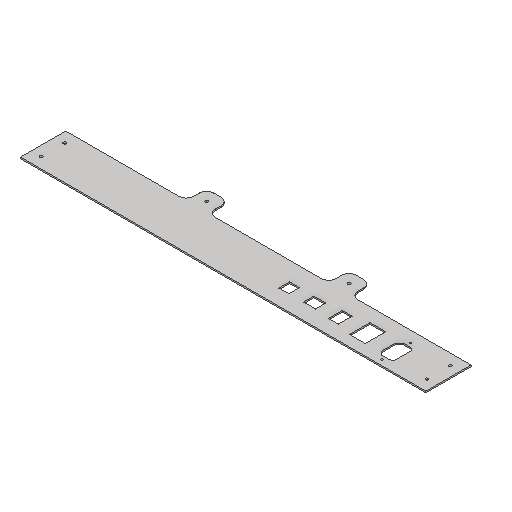
# Autodesk Inventor part: LC_ALU_2mm_Back_Plate
Saved by Autodesk Inventor 2026.1 (Build 301233000, 233)
## iProperties
Created: 2016-06-26
Part Number: LC_ALU_2mm_Back_Plate
Material: Ogólny
Document SubType Name: Modeling
Designer: Andrzej
Density: 1 g/cm^3
Appearance: Obrobione — aluminium
Mass: 72.1532 g
Surface Area: 749.313 cm^2
Volume: 72.1532 cm^3
Author: Andrzej
Autodesk Inventor part; units mm, degrees
ref_plane "YZ Plane" through (0, 0, 0) normal (1, 0, 0) x (0, 1, 0)
ref_plane "XZ Plane" through (0, 0, 0) normal (0, 1, 0) x (-1, 0, 0)
ref_plane "XY Plane" through (0, 0, 0) normal (0, 0, 1) x (1, 0, 0)
sketch "Szkic1" plane through (0, 0, 0) normal (0, 0, 1) x (1, 0, 0)
  line L0 (-89.8533, 62.242) -> (466.1467, 62.242)
  line L1 (466.1467, 62.242) -> (466.1467, 0.242)
  line L2 (466.1467, 0.242) -> (-89.8533, 0.242)
  line L3 (-89.8533, 0.242) -> (-89.8533, 62.242)
  line L4 (75.48, 62.242) -> (105.48, 62.242)
  line L5 (105.48, 62.242) -> (105.48, 90.242)
  line L6 (105.48, 90.242) -> (75.48, 90.242)
  line L7 (75.48, 90.242) -> (75.48, 62.242)
  line L8 (270.8133, 62.242) -> (300.8133, 62.242)
  line L9 (300.8133, 62.242) -> (300.8133, 90.242)
  line L10 (300.8133, 90.242) -> (270.8133, 90.242)
  line L11 (270.8133, 90.242) -> (270.8133, 62.242)
  arc A0 (403.6467, 13.242) -> (407.6467, 17.242) centre (403.6467, 17.242) ccw
  line L12 (407.6467, 17.242) -> (407.6467, 37.242)
  arc A1 (407.6467, 37.242) -> (403.6467, 41.242) centre (403.6467, 37.242) ccw
  line L13 (388.647, 36.242) -> (393.647, 41.242)
  line L14 (388.647, 36.242) -> (388.647, 18.242)
  line L15 (393.647, 13.242) -> (388.647, 18.242)
  line L16 (393.647, 41.242) -> (403.6467, 41.242)
  line L17 (393.647, 13.242) -> (403.6467, 13.242)
  line L18 (393.4399, 41.742) -> (388.147, 36.4491)
  line L19 (388.147, 36.4491) -> (388.147, 18.0348)
  line L20 (388.147, 18.0348) -> (393.4399, 12.742)
  line L21 (393.4399, 12.742) -> (403.6467, 12.742)
  arc A2 (403.6467, 12.742) -> (408.1467, 17.242) centre (403.6467, 17.242) ccw
  line L22 (408.1467, 17.242) -> (408.1467, 37.242)
  arc A3 (408.1467, 37.242) -> (403.6467, 41.742) centre (403.6467, 37.242) ccw
  line L23 (403.6467, 41.742) -> (393.4399, 41.742)
  circle A4 centre (398.6468, 46.742) radius 1.5
  circle A5 centre (398.6467, 7.742) radius 1.5
  line L24 (346.447, 43.242) -> (368.147, 43.242)
  line L25 (368.147, 43.242) -> (368.147, 15.242)
  line L26 (368.147, 15.242) -> (346.447, 15.242)
  line L27 (346.447, 15.242) -> (346.447, 43.242)
  line L28 (276.447, 36.242) -> (292.947, 36.242)
  line L29 (292.947, 36.242) -> (292.947, 22.242)
  line L30 (292.947, 22.242) -> (276.447, 22.242)
  line L31 (276.447, 22.242) -> (276.447, 36.242)
  line L32 (242.947, 36.542) -> (256.447, 36.542)
  line L33 (256.447, 36.542) -> (256.447, 21.942)
  line L34 (256.447, 21.942) -> (242.947, 21.942)
  line L35 (242.947, 21.942) -> (242.947, 36.542)
  line L36 (312.947, 38.742) -> (326.447, 38.742)
  line L37 (326.447, 38.742) -> (326.447, 19.742)
  line L38 (326.447, 19.742) -> (312.947, 19.742)
  line L39 (312.947, 19.742) -> (312.947, 38.742)
  point P0 (90.48, 75.242)
  point P1 (285.8133, 75.242)
  point P2 (-76.3533, 47.242)
  point P3 (452.6467, 47.242)
  point P4 (-76.3533, 15.242)
  point P5 (452.6467, 15.242)
  dimension "d0" = 556
  dimension "d1" = 62
  dimension "d2" = 30
  dimension "d3" = 28
  dimension "d4" = 30
  dimension "d5" = 28
  dimension "d6" = 165.3333
  dimension "d10" = 165.3333
  dimension "d12" = 15
  dimension "d13" = 15
  dimension "d14" = 15
  dimension "d15" = 15
  dimension "d16" = 13.5
  dimension "d17" = 13.5
  dimension "d18" = 15
  dimension "d19" = 15
  dimension "d27" = 13.5
  dimension "d28" = 13.5
  dimension "d29" = 15
  dimension "d30" = 15
  dimension "d42" = 18.9997
  dimension "d43" = 58.5
  dimension "d44" = 28
  dimension "d45" = 21
  dimension "d46" = 14.9997
  dimension "d47" = 4
  dimension "d48" = 4
  dimension "d49" = 14.9997
  dimension "d50" = 5
  dimension "d51" = 5
  dimension "d54" = 0.5
  dimension "d55" = 5.5
  dimension "d56" = 5.5
  dimension "d57" = 8.9999
  dimension "d58" = 9
  dimension "d59" = 3
  dimension "d60" = 3
  dimension "d61" = 10.2068
  dimension "d62" = 9.9997
  dimension "d63" = 9.9997
  dimension "d64" = 10.2068
  dimension "d65" = 28
  dimension "d66" = 21.7
  dimension "d69" = 16.5
  dimension "d71" = 14
  dimension "d72" = 14.6
  dimension "d73" = 13.5
  dimension "d74" = 19
  dimension "d75" = 13.5
  dimension "d76" = 19
  dimension "d77" = 23.5
  dimension "d78" = 26
  dimension "d79" = 25.7
  dimension "d80" = 20
  dimension "d81" = 20
  dimension "d82" = 20
  dimension "d83" = 20
  constraints: 80 end point, 16 parallel, 8 horizontal, 8 point on circle, 7 perpendicular, 6 centre point, 2 coincident, 2 point on line, 7 other
  measures "d0" distance of L1.end L2.end
  measures "d1" distance of L2.end L0.start
  measures "d2" distance of L6.end L5.end
  measures "d3" distance of L5.end L4.end
  measures "d4" distance of L10.end L9.end
  measures "d5" distance of L9.end L8.end
  measures "d6" distance between parallel lines of L3 L7
  measures "d10" distance between parallel lines of L1 L9
  measures "d12" distance from line of L6 point (90.48, 75.242)
  measures "d13" distance from line of L10 point (285.813, 75.242)
  measures "d14" distance from line of L7 point (90.48, 75.242)
  measures "d15" distance from line of L11 point (285.813, 75.242)
  measures "d16" distance from line of L3 point (-76.353, 47.242)
  measures "d17" distance from line of L1 point (452.647, 47.242)
  measures "d18" distance from line of L0 point (-76.353, 47.242)
  measures "d19" distance from line of L0 point (452.647, 47.242)
  measures "d27" distance from line of L3 point (-76.353, 15.242)
  measures "d28" distance from line of L1 point (452.647, 15.242)
  measures "d29" distance from line of L2 point (-76.353, 15.242)
  measures "d30" distance from line of L2 point (452.647, 15.242)
  measures "d42" distance between parallel lines of L12 L14
  measures "d43" distance between parallel lines of L1 L12
  measures "d44" distance between parallel lines of L16 L17
  measures "d45" distance between parallel lines of L0 L16
  measures "d46" distance from line of L14 A1.centre
  measures "d47" distance from line of L16 A1.centre
  measures "d48" distance from line of L17 A0.centre
  measures "d49" distance from line of L14 A0.centre
  measures "d50" horizontal distance of L15.start L15.end
  measures "d51" horizontal distance of L13.start L13.end
  measures "d54" distance between parallel lines of L13 L18
  measures "d55" distance from line of point (398.647, 46.742) L16
  measures "d56" distance from line of L17 point (398.647, 7.742)
  measures "d57" distance from line of L12 point (398.647, 46.742)
  measures "d58" distance from line of L12 point (398.647, 7.742)
  measures "d59" diameter of A4
  measures "d60" diameter of A5
  measures "d61" distance of L23.start L18.start
  measures "d62" distance of L13.end L16.end
  measures "d63" distance of L15.start L17.end
  measures "d64" distance of L20.end L21.end
  measures "d65" distance between parallel lines of L24 L26
  measures "d66" distance between parallel lines of L25 L27
  measures "d69" distance between parallel lines of L29 L31
  measures "d71" distance between parallel lines of L30 L28
  measures "d72" distance between parallel lines of L34 L32
  measures "d73" distance between parallel lines of L33 L35
  measures "d74" distance between parallel lines of L0 L24
  measures "d75" distance of L37.end L38.end
  measures "d76" distance of L36.end L37.end
  measures "d77" distance between parallel lines of L0 L36
  measures "d78" distance between parallel lines of L8 L28
  measures "d79" distance between parallel lines of L0 L32
  measures "d80" distance between parallel lines of L19 L25
  measures "d81" distance between parallel lines of L37 L27
  measures "d82" distance between parallel lines of L29 L39
  measures "d83" distance between parallel lines of L31 L33
extrude "Wyciągnięcie proste1" add sketch "Szkic1" along normal blind 2 contours L0 L1 L2 L3 | L7 L6 L5 L0 | L11 L10 L9 L0 | L17 L15 L14 L13 L16 A1 L12 A0 | L23 A3 L22 A2 L21 L20 L19 L18 | A4 | A5 | L24 L25 L26 L27 | L28 L29 L30 L31 | L32 L33 L34 L35 | L36 L37 L38 L39
fillet "Zaokrąglenie1" radius 10 8 edges at (75.48, 62.242, 1) (75.48, 90.242, 1) (105.48, 90.242, 1) (105.48, 62.242, 1) (270.8133, 62.242, 1) (270.8133, 90.242, 1) (300.8133, 90.242, 1) (300.8133, 62.242, 1)
hole "Otwór1" at (90.48, 75.242, 0) at (285.8133, 75.242, 0) at (-76.3533, 47.242, 0) at (452.6467, 47.242, 0) at (-76.3533, 15.242, 0) at (452.6467, 15.242, 0) direction (0, 0, 1) diameter 4 end through all
extrude "Wyciągnięcie proste2" cut sketch "Szkic1" along normal through all contours L17 L15 L14 L13 L16 A1 L12 A0 | L23 A3 L22 A2 L21 L20 L19 L18 | A4 | A5 | L24 L25 L26 L27 | L28 L29 L30 L31 | L32 L33 L34 L35 | L36 L37 L38 L39
equation "\"d6\" = -0.333333 * d4 + 0.333333 * d0 - 0.333333 * d2"
equation "\"d10\" = d6"
equation "\"d14\" = 0.5 * d2"
equation "\"d15\" = 0.5 * d4"
equation "\"d19\" = d18"
equation "\"d27\" = d16"
equation "\"d28\" = d17"
equation "\"d29\" = d18"
equation "\"d30\" = d19"
